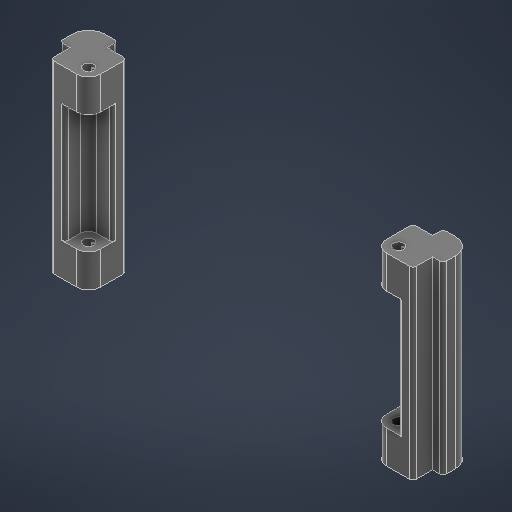
# Autodesk Inventor part: Esquineros Delanteros
Saved by Autodesk Inventor 2026.2 (Build 302298000, 298)
## iProperties
Created: 2026-02-05
Part Number: Esquineros Delanteros
Material: Generic
Document SubType Name: Modeling
Designer: 06aar
Density: 1 g/cm^3
Appearance: Smooth - Black
Author: 06aar
Autodesk Inventor part; units mm, degrees
ref_plane "YZ Plane" through (0, 0, 0) normal (1, 0, 0) x (0, 1, 0)
ref_plane "XZ Plane" through (0, 0, 0) normal (0, 1, 0) x (-1, 0, 0)
ref_plane "XY Plane" through (0, 0, 0) normal (0, 0, 1) x (1, 0, 0)
sketch "Sketch1" plane through (0, 0, 0) normal (0, 1, 0) x (-1, 0, 0)
  line L0 (0, 0) -> (7.6, 0)
  line L1 (7.6, 0) -> (7.6, -4.7)
  line L2 (7.6, -7.2) -> (0, -7.2)
  line L3 (0, -7.2) -> (0, 0)
  line L4 (10.1, -7.2) -> (14.8, -7.2)
  line L5 (14.8, -7.2) -> (14.8, -14.8)
  line L6 (14.8, -14.8) -> (5, -14.8)
  line L7 (0, -9.8) -> (0, -7.2)
  arc A0 (0, -9.8) -> (5, -14.8) centre (5, -9.8) ccw
  circle A1 centre (11.2, -3.6) radius 3.6
  line L8 (7.6, 0) -> (11.2, 0)
  line L9 (14.8, -7.2) -> (14.8, -3.6)
  arc A2 (7.6, -4.7) -> (10.1, -7.2) centre (10.1, -4.7) ccw
  circle A3 centre (11.2, -3.6) radius 1.6
  line L10 (0, 0) -> (3.2, 0)
  line L11 (3.2, 0) -> (3.2, -6)
  line L12 (3.2, -6) -> (0, -6)
  line L13 (0, -6) -> (0, 0)
  line L14 (14.8, -14.8) -> (8.8, -14.8)
  line L15 (8.8, -14.8) -> (8.8, -11.6)
  line L16 (8.8, -11.6) -> (14.8, -11.6)
  line L17 (14.8, -11.6) -> (14.8, -14.8)
  circle A4 centre (11.2, -3.6) radius 1.3
  line L18 (11.2, -3.6) -> (11.2, -5.9)
  circle A5 centre (11.2, -5.9) radius 1
  circle A6 centre (13.1919, -2.45) radius 1
  circle A7 centre (9.2081, -2.45) radius 1
  point P0 (9.9, -14.8)
  point P1 (7.6, -7.4)
  point P2 (8.8, -14.8)
  point P3 (10.6148, -5.0891)
  point P4 (11.7852, -5.0891)
  point P5 (10.203, -2.3486)
  point P6 (9.6178, -3.3623)
  point P7 (12.7822, -3.3623)
  point P8 (12.197, -2.3486)
  dimension "d0" = 5
  dimension "d1" = 7.6
  dimension "d2" = 7.6
  dimension "d3" = 14.8
  dimension "d4" = 14.8
  dimension "d13" = 2.5
  dimension "d14" = 3.2
  dimension "d15" = 2
  dimension "d16" = 3.2
  dimension "d17" = 6
  dimension "d18" = 6
  dimension "d19" = 3.2
  dimension "d24" = 2.6
  dimension "d25" = 2
  dimension "d28" = 360
  constraints: 38 end point, 9 tangent, 8 centre point, 8 parallel, 6 point on circle, 4 horizontal, 4 perpendicular, 3 coincident, 2 point on line, 1 midpoint, 1 vertical, 7 other
  measures "d0" radius of A0
  measures "d1" distance of L0.start L0.end
  measures "d2" distance from line of point (9.9, -14.8) L4
  measures "d3" distance between parallel lines of L6 L0
  measures "d4" distance between parallel lines of L7 L5
  measures "d13" radius of A2
  measures "d14" diameter of A3
  measures "d15" radial gap between concentric circles of A3 A1
  measures "d16" distance between parallel lines of L13 L11
  measures "d17" distance between parallel lines of L0 L12
  measures "d18" distance between parallel lines of L5 L15
  measures "d19" distance between parallel lines of L6 L16
  measures "d24" diameter of A4
  measures "d25" diameter of A5
extrude "Extrusion1" add sketch "Sketch1" along normal blind 28 contours L0 L11 L12 L3 | L0 L1 A2 L4 L5 L16 L15 L6 A0 L7 L3 L12 L11 | L15 L16 L5 L6
extrude "Extrusion2" add sketch "Sketch1" along normal blind 10 contours L8 A1 L1 | A1 L4 A2 L1 | A1 | A1 L9 L4 | A6 A3 | A3 A6 | A5 A3 | A3 L18 A5 | A3 A5 L18 | A7 A3 | A3 A7
extrude "Extrusion3" cut sketch "Sketch1" along normal blind 50 contours L0 L11 L12 L3 | L15 L16 L5 L6
fillet "Fillet1" radius 1 6 edges at (-3.2, 14, 0) (-7.6, 19, 0) (0, 14, -6) (-8.8, 14, -14.8) (-14.8, 14, -11.6) (-14.8, 19, -7.2)
ref_plane "Work Plane1" through (-3.4929, 28, -0.2929) normal (0, 1, 0) x (1, 0, 0)
sketch "Sketch3" plane through (0, 10, 0) normal (0, 1, 0) x (1, 0, 0)
  arc A0 (-12.197, 2.3486) -> (-10.203, 2.3486) centre (-11.2, 3.6) ccw projected
  circle A1 centre (-11.2, 3.6) radius 1.6
  point P0 (0, 0)
  point P1 (-10.203, 2.3486)
  point P2 (-12.197, 2.3486)
  dimension "d33" = 3.2
  constraints: 1 centre point, 1 coincident
  measures "d33" diameter of A1
extrude "Extrusion5" cut sketch "Sketch3" against normal blind 1
ref_plane "Work Plane3" through (0, 5, 0) normal (0, 1, 0) x (1, 0, 0)
mirror "Mirror3" about plane through (0, 5, 0) normal (0, 1, 0) of "Extrusion5"
mirror "Mirror1" about plane through (-3.4929, 28, -0.2929) normal (0, 1, 0)
ref_plane "Work Plane2" through (-58.2232, 0, -10.6) normal (-1, 0, 0) x (0, 0, 1)
mirror "Mirror2" about plane through (-58.2232, 0, -10.6) normal (-1, 0, 0)
body "Solid1"
